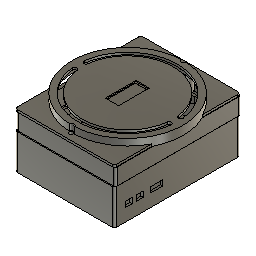
Enclosure v8 (Autodesk Fusion 360 design; units mm, degrees)
Autodesk Fusion 360 part; units mm, degrees
sketch "Sketch2" plane through (0, 0, 0) normal (0, 0, 1) x (1, 0, 0) in component "Component"
  line L0 (-43, 55) -> (43, 55)
  line L1 (43, 55) -> (43, -55)
  line L2 (43, -55) -> (-43, -55)
  line L3 (-43, -55) -> (-43, 55)
  line L4 (-43, 55) -> (43, -55) construction
  line L5 (43, 55) -> (-43, -55) construction
  line L6 (45, -57) -> (-45, -57)
  line L7 (-45, -57) -> (-45, 57)
  line L8 (-45, 57) -> (45, 57)
  line L9 (45, 57) -> (45, -57)
  dimension "d2" = 86
  dimension "d3" = 110
  dimension "d4" = -2
  constraint horizontal L0
  constraint perpendicular L0 L1
  constraint parallel L0 L2
  constraint parallel L1 L3
  constraint coincident L4 origin
  constraint coincident L5 origin
  measures "d2" distance of L0.start L0.end
  measures "d3" distance of L0.end L1.end
extrude "Extrude1" add sketch "Sketch2" along normal blind 1.5 contours L0 L1 L2 L3 | L6 L7 L8 L9 makes body 1 in component "Component"
extrude "Extrude2" add sketch "Sketch2" along normal blind 32 bodies 1 in component "Component"
sketch "Sketch3" plane through (0, 0, 1.5) normal (0, 0, 1) x (-1, 0, 0) in component "Component"
  line L0 (-43, 55) -> (-43, -55)
  line L1 (-43, -55) -> (43, -55)
  line L2 (43, -55) -> (43, 55)
  line L3 (43, 55) -> (-43, 55)
  line L4 (-42.1, -52.75) -> (42.1, -52.75)
  line L5 (42.1, -52.75) -> (42.1, 4.75)
  line L6 (42.1, 4.75) -> (-42.1, 4.75)
  line L7 (-42.1, 4.75) -> (-42.1, -52.75)
  line L8 (-42.1, -52.75) -> (42.1, 4.75) construction
  line L9 (42.1, -52.75) -> (-42.1, 4.75) construction
  line L10 (-37.5, 7.5) -> (37.5, 7.5)
  line L11 (37.5, 7.5) -> (37.5, 52.5)
  line L12 (37.5, 52.5) -> (-37.5, 52.5)
  line L13 (-37.5, 52.5) -> (-37.5, 7.5)
  line L14 (-37.5, 7.5) -> (37.5, 52.5) construction
  line L15 (37.5, 7.5) -> (-37.5, 52.5) construction
  line L16 (0, -55) -> (0, 55) construction
  line L17 (-45, -57) -> (45, -57)
  line L18 (45, 57) -> (-45, 57)
  line L19 (43, 7.5) -> (-43, 7.5)
  line L20 (-35.5, 50.5) -> (-35.5, 9.5)
  line L21 (-35.5, 9.5) -> (35.5, 9.5)
  line L22 (35.5, 9.5) -> (35.5, 50.5)
  line L23 (35.5, 50.5) -> (-35.5, 50.5)
  point P0 (0, -24)
  point P1 (0, 30)
  dimension "d9" = 84.2
  dimension "d10" = 57.5
  dimension "d11" = 45
  dimension "d12" = 75
  dimension "d13" = 33
  dimension "d14" = 27
  dimension "d15" = -2
  constraint horizontal L4
  constraint perpendicular L4 L5
  constraint parallel L4 L6
  constraint parallel L5 L7
  constraint coincident L8 P0
  constraint coincident L9 P0
  constraint horizontal L10
  constraint perpendicular L10 L11
  constraint parallel L10 L12
  constraint parallel L11 L13
  constraint coincident L14 P1
  constraint coincident L15 P1
  constraint midpoint L1 L16.start
  constraint midpoint L3 L16.end
  constraint coincident P0 L16
  constraint coincident P1 L16
  constraint coincident L2 L19.start
  constraint coincident L0 L19.end
  constraint perpendicular L0 L19
  constraint collinear L10 L19
  measures "d9" distance of L4.start L4.end
  measures "d10" distance of L4.start L6.end
  measures "d11" distance of L10.start L12.end
  measures "d12" distance of L11.end L12.end
  measures "d13" distance of P0 L17
  measures "d14" distance of P1 L18
extrude "Extrude3" add sketch "Sketch3" along normal blind 7 contours L10 L11 L12 L13 L19 bodies 1 in component "Component"
extrude "Extrude4" add sketch "Sketch3" along normal blind 9 contours L0 L2 L3 L11 L12 L13 L19 bodies 1 in component "Component"
sketch "Sketch1" plane through (0, 0, 0) normal (0, 1, 0) x (1, 0, 0) in component "Component'"
sketch "Sketch2 (2)" plane through (0, 0, 0) normal (0, 0, 1) x (1, 0, 0) in component "Component'"
  line L0 (42, 28.5) -> (-42, 28.5)
  line L1 (-42, 28.5) -> (-42, -28.5)
  line L2 (-42, -28.5) -> (42, -28.5)
  line L3 (42, -28.5) -> (42, 28.5)
  line L4 (42, 28.5) -> (-42, -28.5) construction
  line L5 (-42, 28.5) -> (42, -28.5) construction
  dimension "d20" = 84
  dimension "d21" = 57
  constraint horizontal L0
  constraint perpendicular L0 L1
  constraint parallel L0 L2
  constraint parallel L1 L3
  constraint coincident L4 origin
  constraint coincident L5 origin
  measures "d20" distance of L0.start L0.end
  measures "d21" distance of L0.start L2.end
extrude "Extrude1'" add sketch "Sketch2 (2)" along normal blind 9.5 separate body makes body 2 in component "Component'"
sketch "Sketch2 (3)" plane through (45, 0, 0) normal (1, 0, 0) x (0, 1, 0)
  line L0 (-57, 0) -> (57, 0)
  line L1 (57, 0) -> (57, 32)
  line L2 (57, 32) -> (-57, 32)
  line L3 (-57, 32) -> (-57, 0)
  line L4 (-7.5, 8.5) -> (-52.5, 8.5) construction
  line L5 (-52.5, 8.5) -> (-52.5, 10.5) construction
  line L6 (-52.5, 10.5) -> (-7.5, 10.5) construction
  line L7 (-7.5, 10.5) -> (-7.5, 8.5)
  line L8 (-40.9, 16.4) -> (-46.9, 16.4)
  line L9 (-46.9, 16.4) -> (-46.9, 11.4)
  line L10 (-46.9, 11.4) -> (-40.9, 11.4)
  line L11 (-40.9, 11.4) -> (-40.9, 16.4)
  line L12 (-40.9, 16.4) -> (-46.9, 11.4) construction
  line L13 (-46.9, 16.4) -> (-40.9, 11.4) construction
  line L14 (-30.9, 16.4) -> (-36.9, 16.4)
  line L15 (-36.9, 16.4) -> (-36.9, 11.4)
  line L16 (-36.9, 11.4) -> (-30.9, 11.4)
  line L17 (-30.9, 11.4) -> (-30.9, 16.4)
  line L18 (-30.9, 16.4) -> (-36.9, 11.4) construction
  line L19 (-36.9, 16.4) -> (-30.9, 11.4) construction
  line L20 (-13, 16.4) -> (-24, 16.4)
  line L21 (-24, 16.4) -> (-24, 11.4)
  line L22 (-24, 11.4) -> (-13, 11.4)
  line L23 (-13, 11.4) -> (-13, 16.4)
  line L24 (-13, 16.4) -> (-24, 11.4) construction
  line L25 (-24, 16.4) -> (-13, 11.4) construction
  line L26 (-43.9, 13.9) -> (-18.5, 13.9) construction
  line L27 (-30, 8.5) -> (-30, 13.9) construction
  point P0 (-43.9, 13.9)
  point P1 (-33.9, 13.9)
  point P2 (-18.5, 13.9)
  point P3 (-30, 13.9)
  dimension "d28" = 5.4
  dimension "d29" = 5
  dimension "d30" = 11
  dimension "d31" = 6
  dimension "d32" = 6
  dimension "d33" = 15.4
  dimension "d34" = 10
  dimension "d35" = 11
  constraint horizontal L8
  constraint perpendicular L8 L9
  constraint parallel L8 L10
  constraint parallel L9 L11
  constraint coincident L12 P0
  constraint coincident L13 P0
  constraint horizontal L14
  constraint perpendicular L14 L15
  constraint parallel L14 L16
  constraint parallel L15 L17
  constraint coincident L18 P1
  constraint coincident L19 P1
  constraint horizontal L20
  constraint perpendicular L20 L21
  constraint parallel L20 L22
  constraint parallel L21 L23
  constraint coincident L24 P2
  constraint coincident L25 P2
  constraint coincident P0 L26.start
  constraint perpendicular L21 L26
  constraint coincident P1 L26
  constraint midpoint L4 L27.start
  constraint perpendicular L4 L27
  constraint coincident L27 P3
  constraint coincident P2 L26.end
  constraint coincident P3 L27.end
  constraint equal L17 L21
  constraint equal L11 L15
  constraint coincident L26 P3
  measures "d28" distance of L27.start P3
  measures "d29" distance of L20.start L22.end
  measures "d30" distance of L20.start L20.end
  measures "d31" distance of L14.start L14.end
  measures "d32" distance of L8.start L8.end
  measures "d33" distance of P1 P2
  measures "d34" distance of P0 P1
  measures "d35" distance of L7 P2
extrude "Extrude5" cut sketch "Sketch2 (3)" against normal blind 9.5 contours L8 L9 L10 L11 | L14 L15 L16 L17 | L20 L21 L22 L23 bodies 1 in component "Component"
sketch "Sketch4" plane through (0, 0, 32) normal (0, 0, 1) x (-1, 0, 0) in component "Component"
  line L0 (-43, 55) -> (43, 55)
  line L1 (43, 55) -> (43, -55)
  line L2 (43, -55) -> (-43, -55)
  line L3 (-43, -55) -> (-43, 55)
  line L4 (45, -57) -> (45, 57)
  line L5 (45, 57) -> (-45, 57)
  line L6 (-45, 57) -> (-45, -57)
  line L7 (-45, -57) -> (45, -57)
  line L8 (41, -53) -> (-41, -53)
  line L9 (41, 53) -> (41, -53)
  line L10 (-41, 53) -> (41, 53)
  line L11 (-41, -53) -> (-41, 53)
  dimension "d57" = 2
  dimension "d58" = 2
  dimension "d59" = 2
  dimension "d60" = 2
  constraint parallel L2 L8
  constraint parallel L1 L9
  constraint parallel L0 L10
  constraint parallel L3 L11
  measures "d57" distance of L3 L11
  measures "d58" distance of L0 L10
  measures "d59" distance of L1 L9
  measures "d60" distance of L2 L8
extrude "Extrude6" add sketch "Sketch4" against normal blind 8 contours L0 L1 L2 L3 bodies 1 in component "Component"
extrude "Extrude7" cut sketch "Sketch4" against normal blind 2 contours L0 L1 L2 L3 bodies 1 in component "Component"
fillet "Fillet1" radius 2 8 edges at (-45, -57, 16) (45, -57, 16) (45, 57, 16) (-45, 57, 16) (43, 55, 12.75) (-43, 55, 12.75) (-43, -55, 17.25) (43, -55, 17.25) on bodies 1 in component "Component"
fillet "Fillet1" radius 2 8 edges at (-41, 53, 27) (-43, 55, 31) (-41, -53, 27) (-43, -55, 31) (41, -53, 27) (43, -55, 31) (41, 53, 27) (43, 55, 31) on bodies 1 in component "Component"
sketch "Sketch5" plane through (0, 0, 30) normal (0, 0, 1) x (-1, 0, 0) in component "Component"
  arc A0 (-43, -53) -> (-41, -55) centre (-41, -53) ccw
  line L0 (-41, -55) -> (41, -55)
  arc A1 (41, -55) -> (43, -53) centre (41, -53) ccw
  line L1 (43, -53) -> (43, 53)
  arc A2 (43, 53) -> (41, 55) centre (41, 53) ccw
  line L2 (41, 55) -> (-41, 55)
  arc A3 (-41, 55) -> (-43, 53) centre (-41, 53) ccw
  line L3 (-43, 53) -> (-43, -53)
  arc A4 (-41, -51) -> (-39, -53) centre (-39, -51) ccw
  line L4 (-41, -51) -> (-41, 51)
  arc A5 (-39, 53) -> (-41, 51) centre (-39, 51) ccw
  line L5 (-39, 53) -> (39, 53)
  arc A6 (41, 51) -> (39, 53) centre (39, 51) ccw
  line L6 (41, 51) -> (41, -51)
  arc A7 (39, -53) -> (41, -51) centre (39, -51) ccw
  line L7 (39, -53) -> (-39, -53)
  line L8 (0, -55) -> (0, 55) construction
  line L9 (43, 0) -> (-43, 0) construction
  circle A8 centre (0, -51) radius 4
  circle A9 centre (-39, 0) radius 4
  circle A10 centre (0, 51) radius 4
  circle A11 centre (39, 0) radius 4
  dimension "d47" = 8
  constraint midpoint L0 L8.start
  constraint midpoint L2 L8.end
  constraint midpoint L1 L9.start
  constraint midpoint L3 L9.end
  constraint coincident L8 A8.centre
  constraint coincident L8.start A8
  constraint coincident L9 A9.centre
  constraint tangent L3 A9
  constraint coincident L8 A10.centre
  constraint coincident L8.end A10
  constraint coincident L9 A11.centre
  constraint coincident L9.start A11
  constraint equal A9 A10
  constraint equal A10 A11
  constraint equal A8 A11
  measures "d47" diameter of A9
extrude "Extrude8" add sketch "Sketch5" against normal blind 6 contours L4 A9 | L7 A8 | L5 A10 | L6 A11 picked at (-38.8353, -0.1123) picked at (0.1116, -49.0114) picked at (0.2592, 49.9416) picked at (38.9525, -0.665) bodies 1 in component "Component"
fillet "Fillet2" radius 2 8 edges at (42.4142, -54.4142, 24) (0, -55, 24) (-42.4142, -54.4142, 24) (-43, 0, 24) (-42.4142, 54.4142, 24) (0, 55, 24) (42.4142, 54.4142, 24) (43, 0, 24) on bodies 1 in component "Component"
sketch "Sketch6" plane through (-45, 0, 0) normal (-1, 0, 0) x (0, -1, 0) in component "Component"
  line L0 (-55, 32) -> (-55, 0)
  line L1 (-55, 0) -> (55, 0)
  line L2 (55, 0) -> (55, 32)
  line L3 (55, 32) -> (-55, 32)
  line L4 (-53, 1.5) -> (-55, 1.5)
  line L5 (-53, 1.5) -> (7.5, 1.5)
  line L6 (7.5, 1.5) -> (-53, 1.5)
  line L7 (-53, 1.5) -> (-55, 1.5)
  line L8 (-16.25, 21.5) -> (-29.25, 21.5)
  line L9 (-29.25, 21.5) -> (-29.25, 13.5)
  line L10 (-29.25, 13.5) -> (-16.25, 13.5)
  line L11 (-16.25, 13.5) -> (-16.25, 21.5)
  line L12 (-16.25, 21.5) -> (-29.25, 13.5) construction
  line L13 (-29.25, 21.5) -> (-16.25, 13.5) construction
  line L14 (-22.75, 1.5) -> (-22.75, 17.5)
  point P0 (-22.75, 17.5)
  dimension "d52" = 16
  dimension "d53" = 13
  dimension "d54" = 8
  constraint horizontal L8
  constraint perpendicular L8 L9
  constraint parallel L8 L10
  constraint parallel L9 L11
  constraint coincident L12 P0
  constraint coincident L13 P0
  constraint midpoint L5 L14.start
  constraint perpendicular L5 L14
  constraint coincident P0 L14.end
  measures "d52" distance of L14.start P0
  measures "d53" distance of L8.start L8.end
  measures "d54" distance of L8.end L9.end
extrude "Extrude9" cut sketch "Sketch6" against normal blind 6.444 contours L8 L9 L10 L11 bodies 1 in component "Component"
fillet "Fillet3" radius 4 6 edges at (3.4641, -53, 27) (-3.4641, -53, 27) (-41, -3.4641, 27) (-41, 3.4641, 27) (41, 3.4641, 27) (41, -3.4641, 27) on bodies 1 in component "Component"
fillet "Fillet3" radius 4 2 edges at (-3.4641, 53, 27) (3.4641, 53, 27) on bodies 1 in component "Component"
sketch "Sketch7" plane through (0, 0, 30) normal (0, 0, 1) x (-1, 0, 0) in component "Component"
  arc A0 (-43, -53) -> (-41, -55) centre (-41, -53) ccw
  line L0 (-41, -55) -> (41, -55)
  arc A1 (41, -55) -> (43, -53) centre (41, -53) ccw
  line L1 (43, -53) -> (43, 53)
  arc A2 (43, 53) -> (41, 55) centre (41, 53) ccw
  line L2 (41, 55) -> (-41, 55)
  arc A3 (-41, 55) -> (-43, 53) centre (-41, 53) ccw
  line L3 (-43, 53) -> (-43, -53)
  arc A4 (-41, -51) -> (-39, -53) centre (-39, -51) ccw
  line L4 (-41, -51) -> (-41, -7.746)
  arc A5 (-38, -3.873) -> (-41, -7.746) centre (-37, -7.746) ccw
  arc A6 (-38, -3.873) -> (-38, 3.873) centre (-39, 0) ccw
  arc A7 (-41, 7.746) -> (-38, 3.873) centre (-37, 7.746) ccw
  line L5 (-41, 7.746) -> (-41, 51)
  arc A8 (-39, 53) -> (-41, 51) centre (-39, 51) ccw
  line L6 (-39, 53) -> (-7.746, 53)
  arc A9 (-3.873, 50) -> (-7.746, 53) centre (-7.746, 49) ccw
  arc A10 (-3.873, 50) -> (3.873, 50) centre (0, 51) ccw
  arc A11 (7.746, 53) -> (3.873, 50) centre (7.746, 49) ccw
  line L7 (7.746, 53) -> (39, 53)
  arc A12 (41, 51) -> (39, 53) centre (39, 51) ccw
  line L8 (41, 51) -> (41, 7.746)
  arc A13 (38, 3.873) -> (41, 7.746) centre (37, 7.746) ccw
  arc A14 (38, 3.873) -> (38, -3.873) centre (39, 0) ccw
  arc A15 (41, -7.746) -> (38, -3.873) centre (37, -7.746) ccw
  line L9 (41, -7.746) -> (41, -51)
  arc A16 (39, -53) -> (41, -51) centre (39, -51) ccw
  line L10 (39, -53) -> (7.746, -53)
  arc A17 (3.873, -50) -> (7.746, -53) centre (7.746, -49) ccw
  arc A18 (3.873, -50) -> (-3.873, -50) centre (0, -51) ccw
  arc A19 (-7.746, -53) -> (-3.873, -50) centre (-7.746, -49) ccw
  line L11 (-7.746, -53) -> (-39, -53)
  point P0 (39, 0)
  point P1 (0, -51)
  point P2 (-39, 0)
  point P3 (0, 51)
  constraint coincident P0 A14.centre
  constraint coincident P1 A18.centre
  constraint coincident P2 A6.centre
  constraint coincident P3 A10.centre
hole "Hole1" at (0, 51, 30) at (-39, 0, 30) at (39, 0, 30) at (0, -51, 30) direction (0, 0, -1) diameter 4.496 depth 8 tip angle 180 bodies 1 in component "Component"
sketch "Sketch1 (2)" plane through (0, 0, 0) normal (0, 0, 1) x (1, 0, 0) in component "Component''"
  line L0 (45, 57) -> (-45, 57)
  line L1 (-45, 57) -> (-45, -57)
  line L2 (-45, -57) -> (45, -57)
  line L3 (45, -57) -> (45, 57)
  line L4 (45, 57) -> (-45, -57) construction
  line L5 (-45, 57) -> (45, -57) construction
  line L6 (-42.2, 54.2) -> (-42.2, -54.2)
  line L7 (-42.2, -54.2) -> (42.2, -54.2)
  line L8 (42.2, -54.2) -> (42.2, 54.2)
  line L9 (42.2, 54.2) -> (-42.2, 54.2)
  dimension "d68" = 90
  dimension "d69" = 114
  dimension "d70" = -2.8
  constraint horizontal L0
  constraint perpendicular L0 L1
  constraint parallel L0 L2
  constraint parallel L1 L3
  constraint coincident L4 origin
  constraint coincident L5 origin
  measures "d68" distance of L1.end L2.end
  measures "d69" distance of L0.start L2.end
extrude "Extrude1''" add sketch "Sketch1 (2)" along normal blind 2 separate body contours L0 L1 L2 L3 | L6 L7 L8 L9 makes body 3 in component "Component''"
fillet "Fillet1'" radius 2 4 edges at (-45, -57, 1) (45, -57, 1) (45, 57, 1) (-45, 57, 1) on bodies 3 in component "Component''"
sketch "Sketch3 (2)" plane through (0, 0, 34) normal (0, 0, 1) x (-1, 0, 0)
  arc A0 (43, -57) -> (45, -55) centre (43, -55) ccw
  line L0 (45, -55) -> (45, 55)
  arc A1 (45, 55) -> (43, 57) centre (43, 55) ccw
  line L1 (43, 57) -> (-43, 57)
  arc A2 (-43, 57) -> (-45, 55) centre (-43, 55) ccw
  line L2 (-45, 55) -> (-45, -55)
  arc A3 (-45, -55) -> (-43, -57) centre (-43, -55) ccw
  line L3 (-43, -57) -> (43, -57)
sketch "Sketch4 (2)" plane through (0, 0, 67.544) normal (0, 0, -1) x (1, 0, 0)
  arc A0 (-42.2, -52.2) -> (-40.2, -54.2) centre (-40.2, -52.2) ccw
  line L0 (-40.2, -54.2) -> (40.2, -54.2)
  arc A1 (40.2, -54.2) -> (42.2, -52.2) centre (40.2, -52.2) ccw
  line L1 (42.2, -52.2) -> (42.2, 52.2)
  arc A2 (42.2, 52.2) -> (40.2, 54.2) centre (40.2, 52.2) ccw
  line L2 (40.2, 54.2) -> (-40.2, 54.2)
  arc A3 (-40.2, 54.2) -> (-42.2, 52.2) centre (-40.2, 52.2) ccw
  line L3 (-42.2, 52.2) -> (-42.2, -52.2)
  circle A4 centre (0, 0) radius 48.5
  circle A5 centre (0, 0) radius 39
  line L4 (0, -54.2) -> (0, 54.2)
  arc A6 (-45, -55) -> (-43, -57) centre (-43, -55) ccw
  line L5 (-43, -57) -> (43, -57)
  arc A7 (43, -57) -> (45, -55) centre (43, -55) ccw
  line L6 (45, -55) -> (45, 55)
  arc A8 (45, 55) -> (43, 57) centre (43, 55) ccw
  line L7 (43, 57) -> (-43, 57)
  arc A9 (-43, 57) -> (-45, 55) centre (-43, 55) ccw
  line L8 (-45, 55) -> (-45, -55)
  circle A10 centre (0, 0) radius 50.5
  dimension "d81" = 97
  dimension "d82" = 78
  dimension "d83" = 2
  constraint coincident A4.centre A5.centre
  constraint midpoint L0 L4.start
  constraint midpoint L2 L4.end
  measures "d81" diameter of A4
  measures "d82" diameter of A5
extrude "Extrude3'" add sketch "Sketch4 (2)" against normal blind 8 contours L3 A4 L8 A10 | L3 A4 L4 A10 | L3 A4 L8 | L3 A4 A5 L4 | A4 L8 A10 | L1 A4 L4 A10 | L3 A4 L8 A10 | L3 A4 L4 A10 | A4 L8 | L1 A4 A5 L4 | L1 A4 L6 A10 | L1 A4 L4 A10 | L1 A4 L6 | A5 L4 | A5 L4 | A4 L6 A10 | L1 A4 L6 A10 | A4 L6 sketch seen with x (1, 0, 0) y (0, 1, 0) z (0, 0, 1) at (0, 0, -67.544) bodies 3 in component "Component''"
extrude "Extrude4'" cut sketch "Sketch4 (2)" along normal blind 2 and the other way blind 6 contours L3 A4 L8 | L3 A4 A5 L4 | A4 L8 | L1 A4 A5 L4 | L1 A4 L6 | A5 L4 | A5 L4 | A4 L6 sketch seen with x (1, 0, 0) y (0, 1, 0) z (0, 0, 1) at (0, 0, -67.544) bodies 3 in component "Component''"
sketch "Sketch5 (2)" plane through (0, 0, 75.544) normal (0, 0, 1) x (-1, 0, 0)
  circle A0 centre (0, 0) radius 50.5
  circle A1 centre (0, 0) radius 43.125 construction
  arc A2 (-44.7886, -5.4994) -> (44.7886, -5.4994) centre (0, 0) ccw
  arc A3 (-40.8185, -5.0119) -> (-44.7886, -5.4994) centre (-42.8036, -5.2556) ccw
  arc A4 (-40.8185, -5.0119) -> (40.8185, -5.0119) centre (0, 0) ccw
  arc A5 (44.7886, -5.4994) -> (40.8185, -5.0119) centre (42.8036, -5.2556) ccw
  arc A6 (-42.8036, -5.2556) -> (42.8036, -5.2556) centre (0, 0) ccw construction
  line L0 (50.5, 0) -> (-51.1033, 0) construction
  line L1 (0, 0) -> (42.8036, -5.2556)
  line L2 (-42.8036, -5.2556) -> (0, 0)
  arc A7 (40.8185, 5.0119) -> (-40.8185, 5.0119) centre (0, 0) ccw
  arc A8 (44.7886, 5.4994) -> (-44.7886, 5.4994) centre (0, 0) ccw
  arc A9 (40.8185, 5.0119) -> (44.7886, 5.4994) centre (42.8036, 5.2556) ccw
  arc A10 (-44.7886, 5.4994) -> (-40.8185, 5.0119) centre (-42.8036, 5.2556) ccw
  dimension "d91" = 86.25
  dimension "d93" = 7
  dimension "d94" = 166
  dimension "d95" = 2
  constraint concentric A0 A1
  constraint tangent A2 A3
  constraint tangent A3 A4
  constraint tangent A4 A5
  constraint tangent A2 A5
  constraint coincident A1 A3.centre
  constraint coincident A1 A5.centre
  constraint coincident A0.centre A1.centre
  constraint coincident A0 L0.start
  constraint horizontal L0
  constraint coincident A5.centre A6.end
  constraint coincident A3.centre A6.start
  constraint symmetric A2.end L0 A8.start
  constraint symmetric A2.start L0 A8.end
  constraint symmetric A3.start L0 A7.end
  constraint symmetric A4.end L0 A7.start
  constraint symmetric A2 L0 A8
  constraint symmetric A3 L0 A10
  constraint symmetric A4 L0 A7
  constraint symmetric A5 L0 A9
  constraint coincident A0.centre L0
  measures "d91" diameter of A1
  measures "d93" angle of L0 L1
  measures "d94" angle of L1 L2
  measures "d95" radius of A3
extrude "Extrude5'" cut sketch "Sketch5 (2)" against normal blind 2 contours A2 A3 A4 A5 | A7 A8 A9 A10 sketch seen with x (1, 0, 0) y (0, 1, 0) z (0, 0, 1) at (0, 0, -67.544) bodies 3 in component "Component''"
sketch "Sketch2 (4)" plane through (0, 0, 2) normal (0, 0, 1) x (-1, 0, 0) in component "Component''"
  arc A0 (-45, -22.9183) -> (45, -22.9183) centre (0, 0) ccw
  line L0 (-45, -22.9183) -> (-45, -55)
  arc A1 (-45, -55) -> (-43, -57) centre (-43, -55) ccw
  line L1 (-43, -57) -> (43, -57)
  arc A2 (43, -57) -> (45, -55) centre (43, -55) ccw
  line L2 (45, -55) -> (45, -22.9183)
  line L3 (0, -57) -> (0, 57)
  line L4 (43, 57) -> (-43, 57)
  circle A3 centre (0, -51) radius 2.5
  circle A4 centre (0, 51) radius 2.5
  point P0 (0, -51)
  point P1 (0, 51)
  dimension "d98" = 102
  dimension "d99" = 51
  dimension "d100" = 5
  dimension "d101" = 5
  constraint midpoint L1 L3.start
  constraint perpendicular L1 L3
  constraint coincident L3.end L4
  constraint coincident L3 P0
  constraint coincident L3 P1
  constraint coincident P0 A3.centre
  constraint coincident P1 A4.centre
  measures "d98" distance of P0 P1
  measures "d99" distance of A0.centre A3.centre
  measures "d100" diameter of A3
  measures "d101" diameter of A4
extrude "Extrude6'" cut sketch "Sketch2 (4)" along normal blind 7 contours A0 L3 A3 | A0 L3 A3 | A0 L3 A3 | A0 L3 A3 | L3 A4 | L3 A4 bodies 3 in component "Component''"
hole "Hole1'" at (0, 51, 2) at (0, -51, 2) direction (0, 0, -1) diameter 3.4 depth 8 tip angle 180 bodies 3 in component "Component''"
sketch "Sketch3 (3)" plane through (0, 0, 6) normal (0, 0, -1) x (1, 0, 0) in component "Component''"
  line L0 (6.5, 19.375) -> (-6.5, 19.375)
  line L1 (-6.5, 19.375) -> (-6.5, -19.375)
  line L2 (-6.5, -19.375) -> (6.5, -19.375)
  line L3 (6.5, -19.375) -> (6.5, 19.375)
  line L4 (6.5, 19.375) -> (-6.5, -19.375) construction
  line L5 (-6.5, 19.375) -> (6.5, -19.375) construction
  line L6 (6, -13.625) -> (-6, -13.625)
  line L7 (-6, -13.625) -> (-6, 14.125)
  line L8 (-6, 14.125) -> (6, 14.125)
  line L9 (6, 14.125) -> (6, -13.625)
  line L10 (6, -13.625) -> (-6, 14.125) construction
  line L11 (-6, -13.625) -> (6, 14.125) construction
  line L12 (0, -19.375) -> (0, 19.375)
  arc A0 (-44.7886, -5.4994) -> (44.7886, -5.4994) centre (0, 0) ccw
  arc A1 (-40.8185, -5.0119) -> (-44.7886, -5.4994) centre (-42.8036, -5.2556) ccw
  arc A2 (-40.8185, -5.0119) -> (40.8185, -5.0119) centre (0, 0) ccw
  arc A3 (44.7886, -5.4994) -> (40.8185, -5.0119) centre (42.8036, -5.2556) ccw
  arc A4 (44.7886, 5.4994) -> (-44.7886, 5.4994) centre (0, 0) ccw
  arc A5 (40.8185, 5.0119) -> (44.7886, 5.4994) centre (42.8036, 5.2556) ccw
  arc A6 (40.8185, 5.0119) -> (-40.8185, 5.0119) centre (0, 0) ccw
  arc A7 (-44.7886, 5.4994) -> (-40.8185, 5.0119) centre (-42.8036, 5.2556) ccw
  arc A8 (0, 48.5) -> (0, -48.5) centre (0, 0) ccw
  arc A9 (0, -48.5) -> (0, 48.5) centre (0, 0) ccw
  point P0 (0, 0.25)
  dimension "d107" = 38.75
  dimension "d108" = 13
  dimension "d109" = 27.75
  dimension "d110" = 12
  dimension "d124" = 5.75
  constraint horizontal L0
  constraint perpendicular L0 L1
  constraint parallel L0 L2
  constraint parallel L1 L3
  constraint coincident L4 A0.centre
  constraint coincident L5 A0.centre
  constraint coincident A0.centre A2.centre
  constraint horizontal L6
  constraint perpendicular L6 L7
  constraint parallel L6 L8
  constraint parallel L7 L9
  constraint coincident L10 P0
  constraint coincident L11 P0
  constraint midpoint L2 L12.start
  constraint midpoint L0 L12.end
  constraint coincident P0 L12
  measures "d107" distance of L0.end L1.end
  measures "d108" distance of L0.start L0.end
  measures "d109" distance of L6.start L8.end
  measures "d110" distance of L7.end L8.end
  measures "d124" distance of L2 L6
extrude "Extrude7'" cut sketch "Sketch3 (3)" against normal blind 2 contours L6 L7 L8 L12 | L6 L8 L9 L12 bodies 3 in component "Component''"
extrude "Extrude8'" cut sketch "Sketch3 (3)" against normal blind 1 contours L0 L2 L3 L6 L8 L9 L12 | L0 L1 L2 L6 L7 L8 L12 bodies 3 in component "Component''"
sketch "Sketch4 (3)" plane through (0, 0, 6) normal (0, 0, -1) x (1, 0, 0) in component "Component''"
  line L0 (-6.5, 19.375) -> (6.5, 19.375)
  line L1 (6.5, 19.375) -> (6.5, -19.375)
  line L2 (6.5, -19.375) -> (-6.5, -19.375)
  line L3 (-6.5, -19.375) -> (-6.5, 19.375)
  line L4 (-8.5, 21.375) -> (8.5, 21.375)
  line L5 (8.5, 21.375) -> (8.5, -21.375)
  line L6 (8.5, -21.375) -> (-8.5, -21.375)
  line L7 (-8.5, -21.375) -> (-8.5, 21.375)
  line L8 (-8.5, 21.375) -> (8.5, -21.375) construction
  line L9 (8.5, 21.375) -> (-8.5, -21.375) construction
  arc A0 (-44.7886, -5.4994) -> (44.7886, -5.4994) centre (0, 0) ccw
  arc A1 (-40.8185, -5.0119) -> (-44.7886, -5.4994) centre (-42.8036, -5.2556) ccw
  arc A2 (-40.8185, -5.0119) -> (40.8185, -5.0119) centre (0, 0) ccw
  arc A3 (44.7886, -5.4994) -> (40.8185, -5.0119) centre (42.8036, -5.2556) ccw
  arc A4 (44.7886, 5.4994) -> (-44.7886, 5.4994) centre (0, 0) ccw
  arc A5 (40.8185, 5.0119) -> (44.7886, 5.4994) centre (42.8036, 5.2556) ccw
  arc A6 (40.8185, 5.0119) -> (-40.8185, 5.0119) centre (0, 0) ccw
  arc A7 (-44.7886, 5.4994) -> (-40.8185, 5.0119) centre (-42.8036, 5.2556) ccw
  arc A8 (0, 48.5) -> (0, -48.5) centre (0, 0) ccw
  arc A9 (0, -48.5) -> (0, 48.5) centre (0, 0) ccw
  dimension "d116" = 2
  dimension "d117" = 2
  constraint horizontal L4
  constraint perpendicular L4 L5
  constraint parallel L4 L6
  constraint parallel L5 L7
  constraint coincident L8 A0.centre
  constraint coincident L9 A0.centre
  constraint coincident A0.centre A2.centre
  measures "d116" distance of L0 L4
  measures "d117" distance of L1 L5
extrude "Extrude9'" add sketch "Sketch4 (3)" along normal blind 3 contours L4 L5 L6 L7 bodies 3 in component "Component''"
sketch "Sketch1 (3)" plane through (0, 0, 0) normal (1, 0, 0) x (0, 1, 0) in component "lcd screen "
  line L0 (19, 6.05) -> (-19, 6.05)
  line L1 (-19, 6.05) -> (-19, -6.05)
  line L2 (-19, -6.05) -> (19, -6.05)
  line L3 (19, -6.05) -> (19, 6.05)
  line L4 (19, 6.05) -> (-19, -6.05) construction
  line L5 (-19, 6.05) -> (19, -6.05) construction
  dimension "d361_1" = 38
  dimension "d362_1" = 12.1
  constraint horizontal L0
  constraint perpendicular L0 L1
  constraint parallel L0 L2
  constraint parallel L1 L3
  constraint coincident L4 origin
  constraint coincident L5 origin
  measures "d361_1" distance of L0.start L0.end
  measures "d362_1" distance of L0.start L2.end
extrude "Extrude1'''" add sketch "Sketch1 (3)" along normal blind 1.25 separate body makes body 4 in component "lcd screen "
sketch "Sketch2 (5)" plane through (1.25, 0, 0) normal (1, 0, 0) x (0, 1, 0) in component "lcd screen "
  line L0 (19, -6.05) -> (19, 6.05)
  line L1 (19, 6.05) -> (-19, 6.05)
  line L2 (-19, 6.05) -> (-19, -6.05)
  line L3 (-19, -6.05) -> (19, -6.05)
  line L4 (-19, 0) -> (-18, 0)
  line L5 (-18, 0) -> (19, 0)
  line L6 (13, 5.875) -> (-14, 5.875)
  line L7 (-14, 5.875) -> (-14, -5.875)
  line L8 (-14, -5.875) -> (13, -5.875)
  line L9 (13, -5.875) -> (13, 5.875)
  line L10 (13, 5.875) -> (-14, -5.875) construction
  line L11 (-14, 5.875) -> (13, -5.875) construction
  point P0 (-0.5, 0)
  dimension "d365_1" = 11.75
  dimension "d366_1" = 27
  dimension "d367_1" = 5
  constraint midpoint L2 L4.start
  constraint perpendicular L2 L4
  constraint midpoint L0 L5.end
  constraint perpendicular L0 L5
  constraint horizontal L6
  constraint perpendicular L6 L7
  constraint parallel L6 L8
  constraint parallel L7 L9
  constraint coincident L10 P0
  constraint coincident L11 P0
  constraint coincident L5 P0
  measures "d365_1" distance of L6.start L8.end
  measures "d366_1" distance of L6.start L6.end
  measures "d367_1" distance of L2 L7
extrude "Extrude2'" add sketch "Sketch2 (5)" along normal blind 2 contours L5 L7 L8 L9 | L5 L6 L7 L9 bodies 4 in component "lcd screen "
sketch "Sketch3 (4)" plane through (1.25, 0, 0) normal (1, 0, 0) x (0, 1, 0) in component "lcd screen "
  line L0 (13, -5.875) -> (-14, -5.875)
  line L1 (-14, -5.875) -> (-14, 5.875)
  line L2 (-14, 5.875) -> (13, 5.875)
  line L3 (13, 5.875) -> (13, -5.875)
  line L4 (19, -6.05) -> (19, 6.05)
  line L5 (19, 6.05) -> (-19, 6.05)
  line L6 (-19, 6.05) -> (-19, -6.05)
  line L7 (-19, -6.05) -> (19, -6.05)
  line L8 (-18.55, 4.875) -> (-17.05, 4.875)
  line L9 (-17.05, 4.875) -> (-17.05, -4.875)
  line L10 (-17.05, -4.875) -> (-18.55, -4.875)
  line L11 (-18.55, -4.875) -> (-18.55, 4.875)
  line L12 (-18.55, 4.875) -> (-17.05, -4.875) construction
  line L13 (-17.05, 4.875) -> (-18.55, -4.875) construction
  line L14 (13, 5.875) -> (19, 5.875)
  line L15 (19, 5.875) -> (19, -5.875)
  line L16 (19, -5.875) -> (13, -5.875)
  line L17 (13, -5.875) -> (13, 5.875)
  line L18 (13, 5.875) -> (19, -5.875) construction
  line L19 (19, 5.875) -> (13, -5.875) construction
  line L20 (-19, 0) -> (19, 0)
  point P0 (-17.8, 0)
  point P1 (16, 0)
  dimension "d370_1" = 1.5
  dimension "d371_1" = 9.75
  dimension "d372_1" = 1.2
  constraint horizontal L8
  constraint perpendicular L8 L9
  constraint parallel L8 L10
  constraint parallel L9 L11
  constraint coincident L12 P0
  constraint coincident L13 P0
  constraint horizontal L14
  constraint perpendicular L14 L15
  constraint parallel L14 L16
  constraint parallel L15 L17
  constraint coincident L18 P1
  constraint coincident L19 P1
  constraint midpoint L6 L20.start
  constraint midpoint L4 L20.end
  constraint coincident P0 L20
  constraint coincident L2.end L3.start
  constraint coincident L4 L15.end
  constraint coincident L0.start L16
  measures "d370_1" distance of L8.start L8.end
  measures "d371_1" distance of L8.start L10.end
  measures "d372_1" distance of P0 L20.start
extrude "Extrude3''" add sketch "Sketch3 (4)" along normal blind 1.5 contours L3 L4 L15 L16 L17 L20 | L3 L4 L14 L15 L17 L20 | L8 L9 L11 L20 | L9 L10 L11 L20 bodies 4 in component "lcd screen "
sketch "Sketch1 (4)" plane through (0, 0, 0) normal (0, 0, 1) x (1, 0, 0) in component "Component'''"
  line L0 (45, 57) -> (-45, 57)
  line L1 (-45, 57) -> (-45, -57)
  line L2 (-45, -57) -> (45, -57)
  line L3 (45, -57) -> (45, 57)
  line L4 (45, 57) -> (-45, -57) construction
  line L5 (-45, 57) -> (45, -57) construction
  line L6 (-42.2, 54.2) -> (-42.2, -54.2)
  line L7 (-42.2, -54.2) -> (42.2, -54.2)
  line L8 (42.2, -54.2) -> (42.2, 54.2)
  line L9 (42.2, 54.2) -> (-42.2, 54.2)
  dimension "d68_1" = 90
  dimension "d69_1" = 114
  dimension "d70_1" = -2.8
  constraint horizontal L0
  constraint perpendicular L0 L1
  constraint parallel L0 L2
  constraint parallel L1 L3
  constraint coincident L4 origin
  constraint coincident L5 origin
  measures "d68_1" distance of L1.end L2.end
  measures "d69_1" distance of L0.start L2.end
extrude "Extrude1''''" add sketch "Sketch1 (4)" along normal blind 15 separate body makes body 5 in component "Component'''"
fillet "Fillet1''" radius 2 4 edges at (-45, -57, 7.5) (45, -57, 7.5) (45, 57, 7.5) (-45, 57, 7.5) on bodies 5 in component "Component'''"
sketch "Sketch2 (6)" plane through (0, 0, 15) normal (0, 0, 1) x (-1, 0, 0) in component "Component'''"
  line L0 (-45, 55) -> (-45, -55)
  arc A0 (-45, -55) -> (-43, -57) centre (-43, -55) ccw
  line L1 (-43, -57) -> (43, -57)
  arc A1 (43, -57) -> (45, -55) centre (43, -55) ccw
  line L2 (45, -55) -> (45, 55)
  line L3 (0, -57) -> (0, 57)
  line L4 (43, 57) -> (-43, 57)
  circle A2 centre (0, -51) radius 2.5
  circle A3 centre (0, 51) radius 2.5
  arc A4 (45, 55) -> (43, 57) centre (43, 55) ccw
  line L5 (43, 57) -> (-43, 57)
  arc A5 (-43, 57) -> (-45, 55) centre (-43, 55) ccw
  line L6 (42.2, -54.2) -> (-42.2, -54.2)
  line L7 (-42.2, -54.2) -> (-42.2, 54.2)
  line L8 (-42.2, 54.2) -> (42.2, 54.2)
  line L9 (42.2, 54.2) -> (42.2, -54.2)
  circle A6 centre (0, 51) radius 6
  circle A7 centre (0, -51) radius 6
  point P0 (0, -51)
  point P1 (0, 51)
  dimension "d98_1" = 102
  dimension "d99_1" = 51
  dimension "d100_1" = 5
  dimension "d101_1" = 5
  constraint midpoint L1 L3.start
  constraint perpendicular L1 L3
  constraint coincident L3.end L4
  constraint coincident L3 P0
  constraint coincident L3 P1
  constraint coincident P0 A2.centre
  constraint coincident P1 A3.centre
  constraint coincident L3.end A6
  constraint coincident L3.start A7
  measures "d98_1" distance of P0 P1
  measures "d99_1" distance of origin A2.centre
  measures "d100_1" diameter of A2
  measures "d101_1" diameter of A3
extrude "Extrude10" add sketch "Sketch2 (6)" against normal blind 15 contours L3 A3 L8 A6 | L3 A3 L8 A6 | L3 A2 L6 A7 | L3 A2 L6 A7 | L3 A3 | L3 A3 | L3 A2 | L3 A2 bodies 5 in component "Component'''"
hole "Hole1''" at (0, 51, 15) at (0, -51, 15) direction (0, 0, -1) diameter 3.9 depth 20 tip angle 180 bodies 5 in component "Component'''"
component "Component" placed x (1, 0, 0) y (0, 1, 0) z (0, 0, 1) at (0, 0, 0)
component "Component'" placed x (1, 0, 0) y (0, 1, 0) z (0, 0, 1) at (0, 23.75, 1.5)
component "Component''" placed x (1, 0, 0) y (0, 1, 0) z (0, 0, 1) at (0, 0, 65.2546)
component "lcd screen " placed x (0, 0, 1) y (0, 1, 0) z (-1, 0, 0) at (0, 0, 68.2546)
component "Component'''" placed x (1, 0, 0) y (0, 1, 0) z (0, 0, 1) at (0, 0, 67.544)
equation "d94 = 180 deg - 14 deg"
equation "d99 = ( 102 / 2 ) * 1 mm"
equation "d99_1 = ( 102 / 2 ) * 1 mm"
